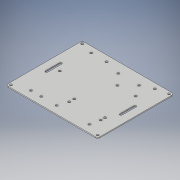
# Autodesk Inventor part: Tier5
Saved by Autodesk Inventor 2018 (Build 220112000, 112)
## iProperties
Created: 2019-03-30
Part Number: Tier5
Material: Generic
Document SubType Name: Modeling
Designer: anirudh
Density: 1 g/cm^3
Appearance: Default
Author: anirudh
Autodesk Inventor part; units mm, degrees
ref_plane "YZ Plane" through (0, 0, 0) normal (1, 0, 0) x (0, 1, 0)
ref_plane "XZ Plane" through (0, 0, 0) normal (0, 1, 0) x (-1, 0, 0)
ref_plane "XY Plane" through (0, 0, 0) normal (0, 0, 1) x (1, 0, 0)
sketch "Sketch1" plane through (0, 0, 0) normal (0, 1, 0) x (-1, 0, 0)
  circle A0 centre (132.6896, -108.9914) radius 1.85
  circle A1 centre (132.6896, 0) radius 1.85
  circle A2 centre (0, 0) radius 1.85
  circle A3 centre (0, -108.9914) radius 1.85
  line L0 (136.4996, -112.8014) -> (-3.81, -112.8014)
  line L1 (-3.81, -112.8014) -> (-3.81, 3.81)
  line L2 (-3.81, 3.81) -> (136.4996, 3.81)
  line L3 (136.4996, 3.81) -> (136.4996, -112.8014)
  dimension "d2" = 3.7
  dimension "d3" = 3.7
  dimension "d4" = 3.7
  dimension "d5" = 3.7
  constraints: 8 end point, 4 centre point, 2 parallel, 1 coincident, 1 horizontal, 1 perpendicular
  measures "d2" diameter of A0
  measures "d3" diameter of A1
  measures "d4" diameter of A2
  measures "d5" diameter of A3
extrude "Extrusion1" add sketch "Sketch1" along normal blind 1.5875
fillet "Fillet1" radius 3.175 4 edges at (3.81, 0.7937, 3.81) (3.81, 0.7937, -112.8014) (-136.4996, 0.7937, -112.8014) (-136.4996, 0.7937, 3.81)
sketch "Sketch2" plane through (0, 1.5875, 0) normal (0, 1, 0) x (1, 0, 0)
  line L0 (-133.3246, -3.81) -> (0.635, -3.81) projected
  circle A0 centre (-94.0054, 7.7978) radius 1.8
  point P0 (0, 0)
  dimension "d16" = 3.6
  constraints: 1 centre point
  measures "d16" diameter of A0
extrude "Extrusion2" cut sketch "Sketch2" against normal blind 1.5875
sketch "Sketch3" plane through (0, 1.5875, 0) normal (0, 1, 0) x (1, 0, 0)
  circle A0 centre (-94.0054, 7.7978) radius 1.8 projected
  circle A1 centre (-20.3454, 7.7978) radius 1.8
  line L0 (0.635, 112.8014) -> (-133.3246, 112.8014) projected
  line L1 (3.81, -0.635) -> (3.81, 109.6264) projected
  circle A2 centre (-34.0106, 97.2566) radius 1.8
  line L2 (-136.4996, 109.6264) -> (-136.4996, -0.635) projected
  circle A3 centre (-113.6904, 103.6828) radius 1.8
  circle A4 centre (-113.6904, 55.7276) radius 1.8
  point P0 (0, 0)
  dimension "d20" = 3.6
  dimension "d30" = 3.6
  dimension "d33" = 3.6
  dimension "d35" = 3.6
  constraints: 4 centre point
  measures "d20" diameter of A1
  measures "d30" diameter of A2
  measures "d33" diameter of A3
  measures "d35" diameter of A4
extrude "Extrusion3" cut sketch "Sketch3" against normal blind 1.5875 contours A1 | A2 | A3 | A4
sketch "Sketch4" plane through (0, 1.5875, 0) normal (0, 1, 0) x (1, 0, 0)
  circle A0 centre (-90.1954, 103.6828) radius 1.8
  circle A1 centre (-90.1954, 103.6828) radius 1.8
  circle A2 centre (-65.7606, 97.2566) radius 1.8
  circle A3 centre (-65.7606, 97.2566) radius 1.8
  circle A4 centre (-17.4244, 104.7496) radius 1.8
  circle A5 centre (-17.4244, 104.7496) radius 1.8
  circle A6 centre (-65.7606, 22.1234) radius 1.8
  circle A7 centre (-65.7606, 22.1234) radius 1.8
  circle A8 centre (-50.4444, 80.5434) radius 1.8
  circle A9 centre (-50.4444, 80.5434) radius 1.8
  circle A10 centre (-22.5044, 80.5434) radius 1.8
  circle A11 centre (-22.5044, 80.5434) radius 1.8
  circle A12 centre (-65.7606, 29.8704) radius 1.8
  circle A13 centre (-65.7606, 29.8704) radius 1.8
  circle A14 centre (-17.4244, 28.4734) radius 1.8
  circle A15 centre (-17.4244, 28.4734) radius 1.8
  circle A16 centre (-17.4244, 22.1234) radius 1.8
  circle A17 centre (-17.4244, 22.1234) radius 1.8
  circle A18 centre (-109.8804, 7.7978) radius 1.8
  circle A19 centre (-109.8804, 7.7978) radius 1.8
  circle A20 centre (-70.5104, 7.7978) radius 1.8
  circle A21 centre (-70.5104, 7.7978) radius 1.8
  line L0 (-136.4996, 109.6264) -> (-136.4996, -0.635) projected
  line L1 (0.635, -3.81) -> (-133.3246, -3.81) projected
  point P0 (0, 0)
  constraints: 22 centre point, 11 coincident
extrude "Extrusion4" cut sketch "Sketch4" against normal blind 1.5875
sketch "Sketch5" plane through (0, 1.5875, 0) normal (0, 1, 0) x (1, 0, 0)
  circle A0 centre (-113.6904, 103.6828) radius 1.8 projected
  arc A1 (-121.39, 66.5353) -> (-124.99, 66.5353) centre (-123.19, 66.5353) ccw
  arc A2 (-124.99, 44.9453) -> (-121.39, 44.9453) centre (-123.19, 44.9453) ccw
  line L0 (-124.99, 44.9453) -> (-124.99, 66.5353)
  line L1 (-121.39, 66.5353) -> (-121.39, 44.9453)
  point P0 (0, 0)
  dimension "d47" = 3.6
  dimension "d49" = 3.6
  constraints: 4 end point, 4 point on circle, 2 centre point, 2 vertical
  measures "d47" diameter of A1
  measures "d49" diameter of A2
extrude "Extrusion5" cut sketch "Sketch5" against normal blind 1.5875 contours L1 A2 L0 A1
ref_plane "Work Plane1" through (-66.3448, 0, 0.635) normal (1, 0, 0) x (0, 0, -1)
mirror "Mirror1" about plane through (-66.3448, 0, 0.635) normal (1, 0, 0) of "Extrusion5"
body "Solid1"
